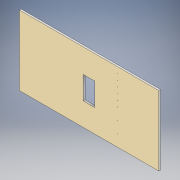
# Autodesk Inventor part: model 2 upper comp front window
Saved by Autodesk Inventor 2017 (Build 210142000, 142)
## iProperties
Created: 2017-06-12
Part Number: model 2 upper comp front window
Material: Generic
Document SubType Name: Modeling
Designer: cas7
Density: 1 g/cm^3
Appearance: Default
Author: cas7
Autodesk Inventor part; units mm, degrees
ref_plane "YZ Plane" through (0, 0, 0) normal (1, 0, 0) x (0, 1, 0)
ref_plane "XZ Plane" through (0, 0, 0) normal (0, 1, 0) x (-1, 0, 0)
ref_plane "XY Plane" through (0, 0, 0) normal (0, 0, 1) x (1, 0, 0)
sketch "Sketch1" plane through (0, 0, 0) normal (0, 0, 1) x (1, 0, 0)
  line L0 (0, 0) -> (1219.2, 0)
  line L1 (1219.2, 0) -> (1219.2, 609.6)
  line L2 (1219.2, 609.6) -> (0, 609.6)
  line L3 (0, 609.6) -> (0, 0)
  line L4 (658.7784, 301.1028) -> (658.7784, 401.1028)
  line L5 (658.7784, 401.1028) -> (558.7784, 401.1028)
  line L6 (558.7784, 401.1028) -> (558.7784, 201.1028)
  line L7 (558.7784, 201.1028) -> (658.7784, 201.1028)
  line L8 (658.7784, 201.1028) -> (658.7784, 301.1028)
  dimension "d0" = 1219.2
  dimension "d1" = 609.6
  dimension "d4" = 100
  dimension "d5" = 100
  dimension "d6" = 200
  dimension "d7" = 100
  constraints: 18 end point, 3 perpendicular, 2 parallel, 1 horizontal, 1 point on line
  measures "d0" distance of L2.end L1.end
  measures "d1" distance of L1.end L0.end
  measures "d4" distance of L4.start L4.end
  measures "d5" distance of L4.end L5.end
  measures "d6" distance of L5.end L6.end
  measures "d7" distance of L6.end L7.end
extrude "Extrusion1" add sketch "Sketch1" along normal blind 15.875
sketch "Sketch2" plane through (0, 0, 15.875) normal (0, 0, 1) x (1, 0, 0)
  line L0 (658.7784, 201.1028) -> (558.7784, 201.1028) projected
  line L1 (558.7784, 201.1028) -> (558.7784, 401.1028) projected
  line L2 (558.7784, 401.1028) -> (658.7784, 401.1028) projected
  line L3 (658.7784, 401.1028) -> (658.7784, 201.1028) projected
  line L4 (0, 0) -> (1219.2, 0) projected
  line L5 (1219.2, 0) -> (1219.2, 609.6) projected
  line L6 (1219.2, 609.6) -> (0, 609.6) projected
  line L7 (0, 609.6) -> (0, 0) projected
sketch "Sketch3" plane through (0, 0, 15.875) normal (0, 0, 1) x (1, 0, 0)
  line L0 (0, 0) -> (859.6758, 0)
  line L1 (0, 0) -> (1219.2, 0) projected
  line L2 (1219.2, 609.6) -> (0, 609.6) projected
  line L3 (859.6758, 0) -> (961.2758, 0) construction
  point P0 (859.6758, 101.6)
  point P1 (859.6758, 203.2)
  point P2 (859.6758, 304.8)
  point P3 (859.6758, 355.6)
  point P4 (859.6758, 406.4)
  point P5 (859.6758, 457.2)
  point P6 (859.6758, 508)
  point P7 (859.6758, 558.8)
  constraints: 4 end point, 1 horizontal, 1 point on line
hole "Hole1" at (859.6758, 101.6, 15.875) at (859.6758, 203.2, 15.875) at (859.6758, 304.8, 15.875) at (859.6758, 355.6, 15.875) at (859.6758, 406.4, 15.875) at (859.6758, 457.2, 15.875) at (859.6758, 508, 15.875) at (859.6758, 558.8, 15.875) direction (0, 0, -1) diameter 3.175 end through all
body "Solid1"
